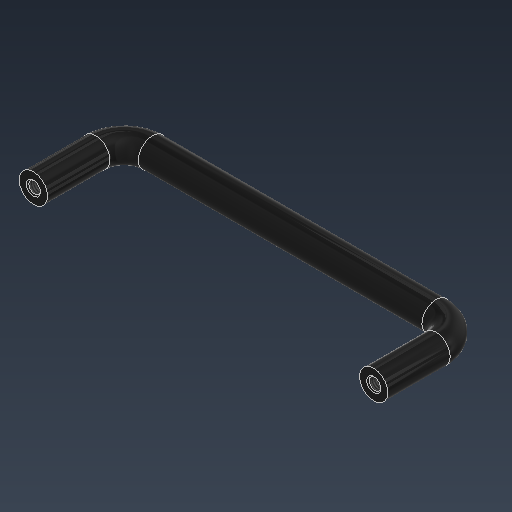
# Autodesk Inventor part: UWANK10-120-27
Saved by Autodesk Inventor 2021 (Build 250183000, 183)
## iProperties
Category: PARTsolutions
Company: MISUMI
Part Number: UWANK10-120-27
Material: 鋼、炭素鋼
Catalog Web Link: www.cadenas.de
Description: UWAN, UWANK, UWANS, UWANA, UWANEA, UWANB, UWANHM, UWANSHM-Round Bar Handles -Dimension Selectable-
Vendor: MISUMI
Document SubType Name: Modeling
Designer: partserver
Manufacturer: MISUMI
Mass: 105.475 g
Surface Area: 59.8288 cm^2
Volume: 13.4363 cm^3
Density: 7.85 g/cm^3
Appearance: 滑らか - 黒
PSOL_IDENT_0: {$CADENAS_DATA\23d-libs\misumi\metric\44_handles_hinges\uwan.prj},239 {VTYP=3D},{NB=UWANK10-120-27},
PSOL_IDENT_1: {LINA=UWANK10-120-27},{NN=UWAN, UWANK, UWANS, UWANA, UWANEA, UWANB, UWANHM, UWANSHM},{DATE=16.06.202
PSOL_IDENT_2: 1 13:36:02},{GEOMDATE=17.02.2014 00:00:00},{VERSION=},{LINEID=10},{WBVAR=TYS,MAT,ST,L,HS,H},{WBNUMER
PSOL_IDENT_3: IC=L,H}  {NB=UWANK10-120-27},{LINA=UWANK10-120-27},{KT=DUMMY},{PN=UWANK10-120-27},{TYPE=UWANK},{TYS=
PSOL_IDENT_4: 1},{TYSALG= '1','Standard','2','Milled' },{MAT=1},{MATALG= '1','12L13 Carbon Steel or 12L14 Carbon S
PSOL_IDENT_5: teel','2','304 Stainless Steel','3','Aluminum Alloy' },{ST=2},{STALG= '1','Chrome Plating','2','Blac
PSOL_IDENT_6: k Oxide' },{D=10},{L=120},{LALG=80,100,110,120,125,160,200,250},{HS=HS},{H=27},{HALG=[27,50]},{HPN=-
PSOL_IDENT_7: 27},{L1=130},{M=5},{AL=2500},{COLOR=0.00,0.00,0.00,0.00},{ML=12.4},{PI=0.8}
NB: UWANK10-120-27
NN: UWAN, UWANK, UWANS, UWANA, UWANEA, UWANB, UWANHM, UWANSHM
NT: Round Bar Handles -Dimension Selectable-
NBSYN: $PN.
LINA: UWANK10-120-27
CATALOG: Misumi
PN: UWANK10-120-27
TYS: Standard
MAT: 12L13 Carbon Steel or 12L14 Carbon Steel
ST: Black Oxide
D: 10
L: 120
HS: Specified
H: 27
L1: 130
M: 5
AL: 2500
SUPPLIER: MISUMI
ARTICLENO: UWANK10-120-27
BOMINFO: UWANK10-120-27
CREATOR: CADENAS GmbH
購入先: ミスミ
在庫数: 0.0
Title: UWANK10-120-27
Author: Cadenas PARTsolutions
Comments: Round Bar Handles -Dimension Selectable-
Autodesk Inventor part; units mm, degrees
sketch "Sketch_1" plane through (0, 0, 0) normal (0, 0, 1) x (1, 0, 0)
  line L0 (0, 0) -> (0, 22)
  line L1 (0, 22) -> (5, 22)
  line L2 (5, 22) -> (5, 0)
  line L3 (5, 0) -> (0, 0)
  line L4 (0, 0) -> (0, 22)
  constraints: 10 end point
revolve "Revolution1" add sketch "Sketch_1" angle 360 about axis through (0, 0, 0) along (0, -1, 0)
sketch "Sketch_2" plane through (0, 22, 0) normal (0, 1, 0) x (1, 0, 0)
  line L0 (10, 10) -> (10, -10)
  circle A0 centre (0, 0) radius 5
  constraints: 2 end point, 1 centre point
revolve "Revolution2" add sketch "Sketch_2" angle 90 about axis through (10, 22, -10) along (0, 0, -1)
sketch "Sketch3" plane through (0, 0, 0) normal (0, -1, 0) x (1, 0, 0)
  point P0 (0, 0)
hole "Hole1" at (0, 0, 0) direction (0, 1, 0) diameter 4.134 depth 12.4 tip angle 120 countersink diameter 5 countersink angle 90 thread size "M5x0.8" class "6H" standard "ISO Metric profile"
sketch "Sketch_4" plane through (0, 0, 0) normal (0, 0, 1) x (1, 0, 0)
  line L0 (110, 32) -> (10, 32)
  line L1 (10, 32) -> (10, 37)
  line L2 (10, 37) -> (110, 37)
  line L3 (110, 37) -> (110, 32)
  line L4 (110, 32) -> (10, 32)
  constraints: 10 end point
revolve "Revolution3" add sketch "Sketch_4" angle 360 about axis through (110, 32, 0) along (1, 0, 0)
sketch "Sketch_6" plane through (0, 22, 0) normal (0, 1, 0) x (1, 0, 0)
  line L0 (110, -10) -> (110, 10)
  circle A0 centre (120, 0) radius 5
  constraints: 2 end point, 1 centre point
revolve "Revolution4" add sketch "Sketch_6" angle 90 about axis through (110, 22, 10) along (0, 0, 1)
sketch "Sketch_5" plane through (0, 0, 0) normal (0, 0, 1) x (1, 0, 0)
  line L0 (120, 0) -> (120, 22)
  line L1 (120, 22) -> (125, 22)
  line L2 (125, 22) -> (125, 0)
  line L3 (125, 0) -> (120, 0)
  line L4 (120, 0) -> (120, 22)
  constraints: 10 end point
revolve "Revolution5" add sketch "Sketch_5" angle 360 about axis through (120, 0, 0) along (0, -1, 0)
sketch "Sketch7" plane through (120, 0, 0) normal (0, -1, 0) x (1, 0, 0)
  point P0 (0, 0)
hole "Hole2" at (120, 0, 0) direction (0, 1, 0) diameter 4.134 depth 12 tip angle 120 countersink diameter 5 countersink angle 90 thread size "M5x0.8" class "6H" standard "ISO Metric profile"
ref_plane "RR_XY" through (60, 32, 0) normal (1, 0, 0) x (0, 0, -1)
ref_plane "RR_YZ" through (60, 32, 0) normal (0, 0, -1) x (0, 1, 0)
ref_plane "RR_ZX" through (60, 32, 0) normal (0, 1, 0) x (1, 0, 0)
ref_plane "U_XY" through (0, 0, 0) normal (0, 1, 0) x (1, 0, 0)
ref_plane "U_YZ" through (0, 0, 0) normal (1, 0, 0) x (0, 0, -1)
ref_plane "U_ZX" through (0, 0, 0) normal (0, 0, -1) x (0, 1, 0)
ref_plane "U1_XY" through (120, 0, 0) normal (0, 1, 0) x (1, 0, 0)
ref_plane "U1_YZ" through (120, 0, 0) normal (1, 0, 0) x (0, 0, -1)
ref_plane "U1_ZX" through (120, 0, 0) normal (0, 0, -1) x (0, 1, 0)
body "Solid1"
